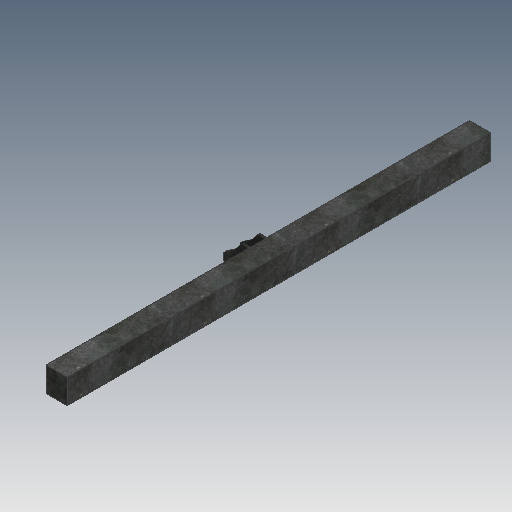
# Autodesk Inventor part: träger hinten mit motorhalterung
Saved by Autodesk Inventor 2020 (Build 240168000, 168)
## iProperties
Created: 2022-01-25
Part Number: träger hinten mit motorhalterung
Material: Stahl
Document SubType Name: Modeling
Designer: mike8
Density: 7.85 g/cm^3
Appearance: Platte
Mass: 4984.26 g
Surface Area: 845.999 cm^2
Volume: 634.937 cm^3
Author: mike8
Autodesk Inventor part; units mm, degrees
ref_plane "YZ Plane" through (0, 0, 0) normal (1, 0, 0) x (0, 1, 0)
ref_plane "XZ Plane" through (0, 0, 0) normal (0, 1, 0) x (-1, 0, 0)
ref_plane "XY Plane" through (0, 0, 0) normal (0, 0, 1) x (1, 0, 0)
sketch "Skizze1" plane through (0, 0, 0) normal (0, 0, 1) x (1, 0, 0)
  line L0 (-65.5041, 0) -> (25.4959, 0) projected
  line L1 (0, -27.5001) -> (0, 21.4999) projected
  line L2 (-17.5041, 14.4999) -> (12.4959, 14.4999)
  line L3 (12.4959, 14.4999) -> (12.4959, -20.5001)
  line L4 (12.4959, -20.5001) -> (-17.5041, -20.5001)
  line L5 (-17.5041, -20.5001) -> (-17.5041, 14.4999)
  point P0 (0, 0)
  dimension "d0" = 30
  dimension "d1" = 35
  constraints: 8 end point, 2 parallel, 1 horizontal, 1 perpendicular
  measures "d0" distance of L2.start L2.end
  measures "d1" distance of L4.end L2.start
extrude "Extrusion1" add sketch "Skizze1" along normal blind 600
sketch "Skizze2" plane through (-17.5041, -20.5001, 0) normal (-1, 0, 0) x (0, 0, 1)
  line L0 (0, 0) -> (600, 0) projected
  line L1 (287, 35) -> (290, 35)
  line L2 (290, 35) -> (290, 0)
  line L3 (290, 0) -> (287, 0)
  line L4 (287, 0) -> (287, 35)
  line L5 (0, 35) -> (600, 35) projected
  line L6 (310, 35) -> (313, 35)
  line L7 (313, 35) -> (313, 0)
  line L8 (313, 0) -> (310, 0)
  line L9 (310, 0) -> (310, 35)
  line L10 (600, 35) -> (600, 0) projected
  point P0 (0, 20.5001)
  point P1 (310, 0)
  point P2 (313, 0)
  point P3 (287, 0)
  dimension "d4" = 287
  dimension "d5" = 3
  dimension "d6" = 20
  dimension "d7" = 3
  dimension "d10" = 35
  constraints: 16 end point, 4 parallel, 3 point on line, 2 horizontal, 2 perpendicular
  measures "d4" distance between parallel lines of L10 L7
  measures "d5" distance between parallel lines of L7 L9
  measures "d6" distance between parallel lines of L9 L2
  measures "d7" distance between parallel lines of L2 L4
  measures "d10" distance of L3.end L1.start
extrude "Extrusion2" add sketch "Skizze2" along normal blind 35 contours L4 L1 L2 L0 | L9 L5 L7 L0
sketch "Skizze3" plane through (-17.5041, -20.5001, 313) normal (0, 0, 1) x (1, 0, 0)
  line L0 (0, 35) -> (-35, 35) projected
  line L1 (-10, 35) -> (-20, 22.6396)
  line L2 (-20, 22.6396) -> (-35, 12.5)
  line L3 (-35, 12.5) -> (-35, 35)
  line L4 (-35, 35) -> (-10, 35)
  point P0 (17.5041, 20.5001)
  dimension "d11" = 25
  dimension "d12" = 15
  dimension "d13" = 22.5
  constraints: 8 end point, 2 perpendicular, 2 point on line
  measures "d11" distance of L0.end L4.end
  measures "d12" horizontal distance of L1.end L2.end
  measures "d13" distance of L2.end L0.end
extrude "Extrusion3" cut sketch "Skizze3" against normal blind 50
fillet "Rundung1" radius 2 4 edges at (-52.5041, -8.0001, 288.5) (-52.5041, -8.0001, 311.5) (-52.5041, -20.5001, 288.5) (-52.5041, -20.5001, 311.5)
sketch "Skizze4" plane through (-17.5041, -20.5001, 313) normal (0, 0, 1) x (1, 0, 0)
  line L0 (-35, 2) -> (-35, 11.4379) projected
  line L1 (0, 0) -> (-33, 0) projected
  point P0 (17.5041, 20.5001)
  point P1 (-27, 8)
  dimension "d17" = 8
  dimension "d18" = 8
  measures "d17" distance from line of L0 point (-27, 8)
  measures "d18" distance from line of L1 point (-27, 8)
hole "Bohrung1" at (-44.5041, -12.5001, 313) direction (0, 0, -1) diameter 3 end through all
sketch "Skizze5" plane through (-17.5041, -20.5001, 600) normal (-1, 0, 0) x (0, 0, 1)
  line L0 (0, 35) -> (0, 0) projected
  line L1 (-600, 35) -> (-600, 0) projected
  line L2 (-600, 35) -> (-313, 35) projected
  line L3 (-287, 35) -> (0, 35) projected
  point P0 (-600, 20.5001)
  point P1 (-585, 17.5)
  point P2 (-15, 17.5)
  dimension "d26" = 15
  dimension "d27" = 15
  dimension "d28" = 17.5
  dimension "d29" = 17.5
  measures "d26" distance from line of point (-15, 17.5) L0
  measures "d27" distance from line of L1 point (-585, 17.5)
  measures "d28" distance from line of L2 point (-585, 17.5)
  measures "d29" distance from line of L3 point (-15, 17.5)
hole "Bohrung2" at (-17.5041, -3.0001, 15) at (-17.5041, -3.0001, 585) direction (1, 0, 0) diameter 3 depth 30 tip angle 118
